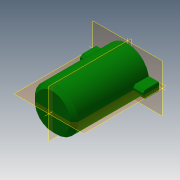
# Autodesk Inventor part: HbThumbLockButton01
Saved by Autodesk Inventor 2015 SP1 (Build 190203100, 203)
## iProperties
Created: 2015-09-12
Part Number: HbThumbLockButton01
Material: ABS プラスチック
Document SubType Name: Modeling
Designer: Yamaura
Density: 1.06 g/cm^3
Appearance: 濃い緑
Author: Yamaura
Autodesk Inventor part; units mm, degrees
sketch "スケッチ1" plane through (0, 0, 0) normal (0, 0, 1) x (1, 0, 0)
  circle A0 centre (0, 0) radius 5.5
  dimension "d0" = 11
  constraints: 1 centre point, 1 coincident
  measures "d0" diameter of A0
extrude "押し出し1" add sketch "スケッチ1" along normal blind 19
sketch "スケッチ3" plane through (0, 0, 0) normal (0, 0, 1) x (1, 0, 0)
  point P0 (0, 0)
sketch "スケッチ4" plane through (0, 0, 0) normal (0, 0, 1) x (1, 0, 0)
  line L0 (-7.9373, -1) -> (7.9373, -1)
  line L1 (7.9373, 1) -> (-7.9373, 1)
  line L2 (-8, -1) -> (8, 1) construction
  line L3 (8, -1) -> (-8, 1) construction
  arc A0 (7.9373, -1) -> (7.9373, 1) centre (0, 0) ccw
  arc A1 (-7.9373, 1) -> (-7.9373, -1) centre (0, 0) ccw
  dimension "d6" = 2
  dimension "d7" = 16
  constraints: 8 end point, 4 point on circle, 2 centre point, 2 midpoint, 1 coincident, 1 horizontal, 1 parallel
  measures "d6" distance of L3.start L2.end
  measures "d7" distance of L2.end L3.end
extrude "押し出し3" add sketch "スケッチ4" along normal blind 4
sketch "スケッチ2" plane through (0, 0, 0) normal (0, 0, 1) x (1, 0, 0)
  circle A0 centre (0, 0) radius 3.5
  dimension "d3" = 7
  constraints: 1 centre point, 1 coincident
  measures "d3" diameter of A0
extrude "押し出し2" cut sketch "スケッチ2" along normal blind 3.5
chamfer "面取り1" distance 0.5 angle 45 4 edges at (6.6728, -1, 4) (-6.6728, -1, 4) (-6.6728, 1, 4) (6.6728, 1, 4)
sketch "スケッチ5" plane through (0, 0, 3.5) normal (0, 0, -1) x (-1, 0, 0)
  circle A0 centre (0, 0) radius 2
  dimension "d13" = 4
  constraints: 1 centre point, 1 coincident
  measures "d13" diameter of A0
extrude "押し出し4" add sketch "スケッチ5" along normal blind 1.5
chamfer "面取り2" distance 1 angle 45 1 edges at (-5.5, 0, 19)
